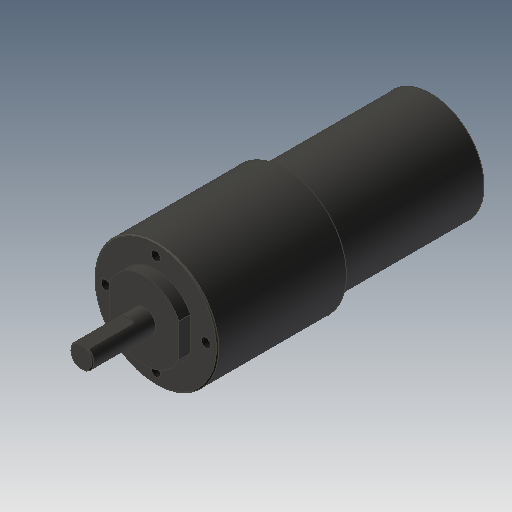
# Autodesk Inventor part: RS385PH_Geared_Motor
Saved by Autodesk Inventor 2019.4 (Build 234330000, 330)
## iProperties
Created: 2018-05-19
Part Number: RS385PH_Geared_Motor
Material: 鋼、鍛鋼
Document SubType Name: Modeling
Designer: AzLIer
Density: 7.85 g/cm^3
Appearance: 鋼
Mass: 240 g
Surface Area: 129.852 cm^2
Volume: 91.3709 cm^3
Author: AzLIer
Autodesk Inventor part; units mm, degrees
ref_plane "YZ Plane" through (0, 0, 0) normal (1, 0, 0) x (0, 1, 0)
ref_plane "XZ Plane" through (0, 0, 0) normal (0, 1, 0) x (-1, 0, 0)
ref_plane "XY Plane" through (0, 0, 0) normal (0, 0, 1) x (1, 0, 0)
sketch "スケッチ1" plane through (0, 0, 0) normal (0, 0, 1) x (1, 0, 0)
  circle A0 centre (0, 0) radius 3
  dimension "d0" = 6
  constraints: 1 centre point, 1 coincident
  measures "d0" diameter of A0
extrude "押し出し1" add sketch "スケッチ1" along normal blind 16.3
sketch "スケッチ2" plane through (0, 0, 16.3) normal (0, 0, 1) x (1, 0, 0)
  circle A0 centre (0, 0) radius 3 projected
  line L0 (-1.6583, 2.5) -> (1.6583, 2.5)
  dimension "d3" = 5.5
  constraints: 2 end point, 2 point on circle, 1 horizontal
extrude "押し出し2" cut sketch "スケッチ2" against normal blind 12 contours L0 A0 picked at (-0.1169, 2.6598)
chamfer "面取り1" distance 0.3 angle 45 2 edges at (-1.4186, -2.6434, 16.3) (2.6434, 1.4186, 16.3)
sketch "スケッチ3" plane through (0, 0, 0) normal (0, 0, -1) x (-1, 0, 0)
  circle A0 centre (0, 0) radius 10
  dimension "d9" = 20
  constraints: 1 centre point, 1 coincident
  measures "d9" diameter of A0
extrude "押し出し3" add sketch "スケッチ3" along normal blind 3
sketch "スケッチ4" plane through (0, 0, -3) normal (0, 0, -1) x (-1, 0, 0)
  circle A0 centre (0, 0) radius 10 projected
  line L0 (9, 4.3589) -> (9, -4.3589)
  line L1 (-9, 4.3589) -> (-9, -4.3589)
  dimension "d12" = 18
  constraints: 4 end point, 4 point on circle, 2 parallel, 1 vertical
  measures "d12" distance between parallel lines of L1 L0
extrude "押し出し4" cut sketch "スケッチ4" against normal blind 3 contours A0 L0 | L1 A0
sketch "スケッチ5" plane through (0, 0, -3) normal (0, 0, -1) x (-1, 0, 0)
  circle A0 centre (0, 0) radius 16
  dimension "d15" = 32
  constraints: 1 centre point, 1 coincident
  measures "d15" diameter of A0
extrude "押し出し5" add sketch "スケッチ5" along normal blind 33.4
chamfer "面取り2" distance 0.3 angle 45 1 edges at (16, 0, -3)
sketch "スケッチ6" plane through (0, 0, -3) normal (0, 0, 1) x (1, 0, 0)
  arc A0 (9, 4.3589) -> (-9, 4.3589) centre (0, 0) ccw projected
  point P0 (0, 13)
  point P1 (-13, 0)
  point P2 (0, -13)
  point P3 (13, 0)
  dimension "d21" = 13
  dimension "d24" = 360
  constraints: 1 vertical alignment, 5 other
  measures "d21" distance of A0.centre point (0, 13)
hole "穴1" at (0, 13, -3) at (-13, 0, -3) at (0, -13, -3) at (13, 0, -3) direction (0, 0, -1) diameter 2.459 depth 6 tip angle 118 thread size "M3x0.5" class "6H" standard "ANSI Metric M Profile"
sketch "スケッチ7" plane through (0, 0, -36.4) normal (0, 0, -1) x (-1, 0, 0)
  circle A0 centre (0, 0) radius 13.85
  dimension "d33" = 27.7
  constraints: 1 centre point, 1 coincident
  measures "d33" diameter of A0
extrude "押し出し6" add sketch "スケッチ7" along normal blind 37.8
